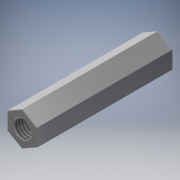
# Autodesk Inventor part: 09-0001
Saved by Autodesk Inventor 2017.1 (Build 211199000, 199)
## iProperties
Category: Standoff Spacer Service Pack
Company: Autodesk Inc.
Created: 2014-11-30
Part Number: 09-0001
Material: Aluminum 6061
Document SubType Name: Modeling
Designer: Matrix
Density: 2.7 g/cm^3
Appearance: Aluminum - Polished
Catalog Web Link: http://matrixrobotics.com/
Vendor: Matrix
Author: Autodesk Inc.
Autodesk Inventor part; units mm, degrees
ref_plane "YZ Plane" through (0, 0, 0) normal (1, 0, 0) x (0, 1, 0)
ref_plane "XZ Plane" through (0, 0, 0) normal (0, 1, 0) x (-1, 0, 0)
ref_plane "XY Plane" through (0, 0, 0) normal (0, 0, 1) x (1, 0, 0)
sketch "Sketch1" plane through (0, 0, 0) normal (0, 1, 0) x (-1, 0, 0)
  line L0 (-3.5, -2.0207) -> (-3.5, 2.0207)
  line L1 (-3.5, 2.0207) -> (0, 4.0415)
  line L2 (0, 4.0415) -> (3.5, 2.0207)
  line L3 (3.5, 2.0207) -> (3.5, -2.0207)
  line L4 (3.5, -2.0207) -> (0, -4.0415)
  line L5 (0, -4.0415) -> (-3.5, -2.0207)
  point P0 (0, 0)
  point P1 (0, 0)
  dimension "d0" = 7
  constraints: 12 end point, 1 coincident, 1 vertical, 13 other
  measures "d0" distance between parallel lines of L0 L3
extrude "Extrusion1" add sketch "Sketch1" against normal blind 32
chamfer "Chamfer1" distance 0.1 angle 45 12 edges at (-1.75, -32, 3.0311) (1.75, -32, 3.0311) (3.5, -32, 0) (1.75, -32, -3.0311) (-1.75, -32, -3.0311) (-3.5, -32, 0) (1.75, 0, 3.0311) (-1.75, 0, 3.0311) (-3.5, 0, 0) (-1.75, 0, -3.0311) (1.75, 0, -3.0311) (3.5, 0, 0)
sketch "Sketch2" plane through (0, -32, 0) normal (0, -1, 0) x (1, 0, 0)
  circle A0 centre (0, 0) radius 2
  dimension "d6" = 4
  constraints: 1 centre point, 1 coincident
  measures "d6" diameter of A0
extrude "Extrusion2" cut sketch "Sketch2" against normal blind 8
sketch "Sketch3" plane through (0, 0, 0) normal (0, 1, 0) x (1, 0, 0)
  circle A0 centre (0, 0) radius 2
  dimension "d9" = 4
  constraints: 1 centre point, 1 coincident
  measures "d9" diameter of A0
extrude "Extrusion3" cut sketch "Sketch3" against normal blind 8
chamfer "Chamfer2" distance 0.2 angle 45 2 edges at (-2, 0, 0) (-2, -32, 0)
thread "Thread1" size "M4x0.7" class "6H" standard "ANSI Metric M Profile" full length
thread "Thread2" size "M4x0.7" class "6H" standard "ANSI Metric M Profile" full length
body "Solid1"
